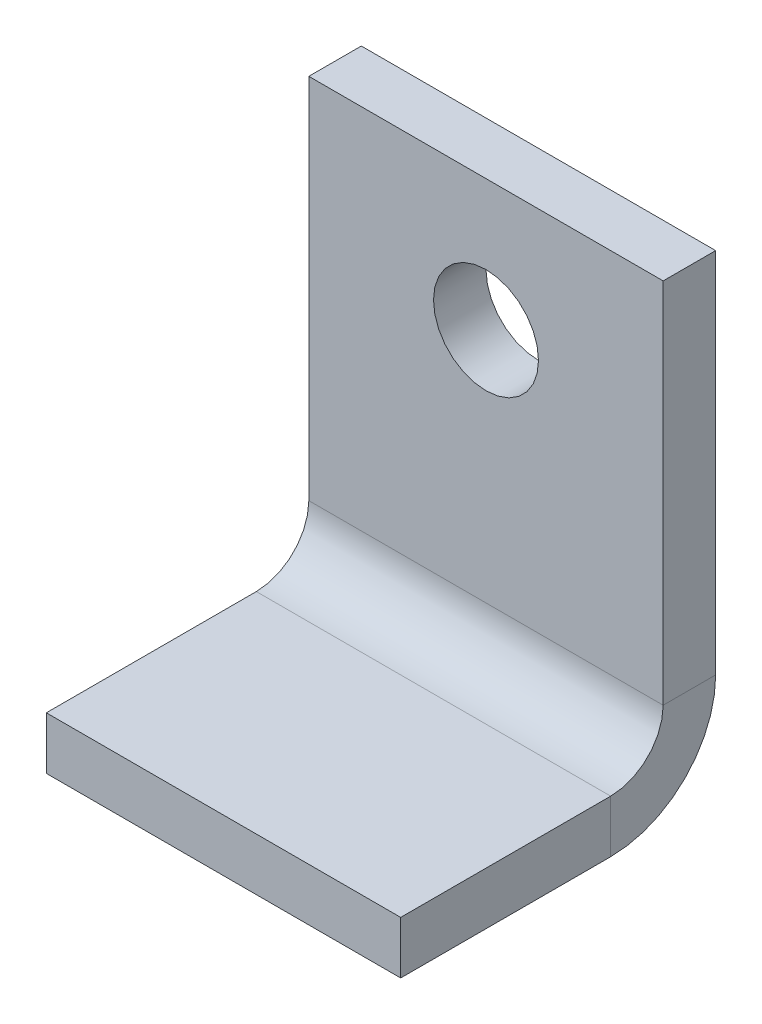
# Autodesk Inventor part: BackWheelMountingPlate
Saved by Autodesk Inventor 2022.2 (Build 262287000, 287)
## iProperties
Created: 2022-03-25
Part Number: BackWheelMountingPlate
Material: Generic
Document SubType Name: Sheet Metal
Designer: Finn Oriwohl
Density: 1 g/cm^3
Sheet Metal Rule: Default_mm
Appearance: Default
Author: Finn Oriwohl
Autodesk Inventor part; units mm, degrees
ref_plane "YZ Plane" through (0, 0, 0) normal (1, 0, 0) x (0, 1, 0)
ref_plane "XZ Plane" through (0, 0, 0) normal (0, 1, 0) x (-1, 0, 0)
ref_plane "XY Plane" through (0, 0, 0) normal (0, 0, 1) x (1, 0, 0)
ref_plane "Work Plane1" through (-238.4764, 144.082, 198.5771) normal (0, 1, 0) x (-1, 0, 0)
ref_plane "Work Plane2" through (-231.6014, 144.082, 198.5771) normal (0, 1, 0) x (1, 0, 0)
sketch "Sketch1" plane through (-231.6014, 144.082, 198.5771) normal (0, 1, 0) x (1, 0, 0)
  line L0 (-13.5, 2) -> (0, 2) projected
  line L1 (-13.5, 0) -> (-13.5, 2) projected
  line L2 (0, 0) -> (-13.5, 0) projected
  line L3 (0, 0) -> (0, 2) projected
  line L4 (-13.5, 0) -> (0, 0)
  line L5 (0, 0) -> (0, 12)
  line L6 (0, 12) -> (-13.5, 12)
  line L7 (-13.5, 12) -> (-13.5, 0)
  point P0 (231.6014, 198.5771)
  point P1 (0, 2)
  dimension "d0" = 12
  constraints: 8 end point, 2 parallel, 1 horizontal, 1 perpendicular
  measures "d0" distance of L5.end L4.end
extrude "Extrusion1" add sketch "Sketch1" along normal blind 2
ref_plane "Work Plane3" through (-238.3514, 162.082, 188.5771) normal (0, 1, 0) x (1, 0, 0)
sketch "Sketch2" plane through (-238.3514, 162.082, 188.5771) normal (0, 1, 0) x (1, 0, 0)
  line L0 (-10, 0) -> (10, 0)
  point P0 (238.3514, 188.5771)
  constraints: 2 end point, 1 horizontal
sketch "Sketch3" plane through (-245.1014, 144.082, 188.5771) normal (0, 0, -1) x (-1, 0, 0)
  line L0 (-13.5, 0) -> (0, 0)
  line L1 (0, 0) -> (0, 18)
  line L2 (0, 18) -> (-13.5, 18)
  line L3 (-13.5, 18) -> (-13.5, 0)
  constraints: 6 end point, 1 horizontal, 1 perpendicular, 1 vertical
edge flange "Flange1" height 18 angle 90 thickness 2 bend radius 2 thickness toward (0, 0, -1) relief straight relief width 2 relief depth 1 edges at (-238.3514, 146.082, 186.5771) wall of the first edge with corners at (-231.6014, 144.082, 188.5771) (-245.1014, 144.082, 188.5771) (-245.1014, 162.082, 188.5771) (-231.6014, 162.082, 188.5771)
bend "Bend1"
corner "Corner1"
sketch "Sketch4" plane through (-245.1014, 162.082, 188.5771) normal (0, 0, 1) x (1, 0, 0)
  circle A0 centre (6.75, -5) radius 2
  line L0 (13.5, 0) -> (0, 0) projected
  line L1 (6.75, 0) -> (6.75, -8.3247) construction
  point P0 (245.1014, -162.082)
  point P1 (6.75, -3)
  dimension "d14" = 4
  dimension "d15" = 3
  constraints: 2 end point, 2 midpoint, 2 point on line, 1 vertical, 1 vertical alignment, 2 other
  measures "d15" distance of point (6.75, 0) point (6.75, -3)
extrude "Extrusion2" cut sketch "Sketch4" against normal through all
equation "\"d3\" = Thickness"
equation "\"d4\" = BendReliefWidth"
equation "\"d5\" = BendReliefDepth"
equation "\"d6\" = MinimumRemnant"
equation "\"d7\" = TransitionRadius"
equation "\"d10\" = BendRadius"
equation "\"d11\" = CornerReliefSize"
equation "\"d12\" = GapSize"
equation "\"d13\" = JacobiRadiusSize"
equation "\"BendRadius\" = Thickness"
equation "\"BendReliefWidth\" = Thickness"
equation "\"BendReliefDepth\" = 0.5 * Thickness"
equation "\"CornerReliefSize\" = 4 * Thickness"
equation "\"MinimumRemnant\" = 2 * Thickness"
equation "\"TransitionRadius\" = BendRadius"
equation "\"JacobiRadiusSize\" = BendRadius"
equation "\"GapSize\" = Thickness"
equation "\"Thickness\" = 2"
body "Solid1"
